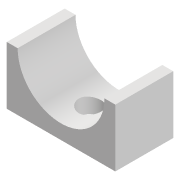
# Autodesk Inventor part: Tube_adaptor_2
Saved by Autodesk Inventor 2022 (Build 260153000, 153)
## iProperties
Created: 2022-06-09
Part Number: Tube_adaptor_2
Material: Generic
Document SubType Name: Modeling
Designer: dell
Density: 1 g/cm^3
Appearance: Default
Author: dell
Autodesk Inventor part; units mm, degrees
ref_plane "YZ Plane" through (0, 0, 0) normal (1, 0, 0) x (0, 1, 0)
ref_plane "XZ Plane" through (0, 0, 0) normal (0, 1, 0) x (-1, 0, 0)
ref_plane "XY Plane" through (0, 0, 0) normal (0, 0, 1) x (1, 0, 0)
sketch "Sketch1" plane through (0, 0, 0) normal (0, 0, 1) x (1, 0, 0)
  circle A0 centre (0, 0) radius 6
  line L0 (-7.5, 0) -> (7.5, 0)
  line L1 (7.5, 0) -> (7.5, -8)
  line L2 (7.5, -8) -> (-7.5, -8)
  line L3 (-7.5, -8) -> (-7.5, 0)
  point P0 (6, 0)
  point P1 (-6, 0)
  point P2 (6, 0)
  point P3 (-6, 0)
  dimension "d0" = 12
  dimension "d1" = 2
  dimension "d2" = 7.5
  dimension "d3" = 7.5
  constraints: 8 end point, 2 parallel, 1 centre point, 1 coincident, 1 horizontal, 1 midpoint, 1 perpendicular
  measures "d0" diameter of A0
  measures "d1" distance edge to line of A0 L2
  measures "d2" distance from line of point (0, 0) L1
  measures "d3" distance from line of point (0, 0) L3
extrude "Extrusion1" add sketch "Sketch1" along normal blind 8 contours L0 L1 L2 L3 A0
sketch "Sketch2" plane through (-7.5, -8, 0) normal (0, -1, 0) x (1, 0, 0)
  line L0 (0, 0) -> (15, 0) projected
  line L1 (15, 0) -> (15, 8) projected
  line L2 (0, 8) -> (15, 8) projected
  line L3 (0, 0) -> (0, 8) projected
  line L4 (0, 8) -> (15, 8) construction
  line L5 (15, 0) -> (0, 8) construction
  line L6 (0, 0) -> (15, 0) construction
  line L7 (15, 8) -> (0, 0) construction
  circle A0 centre (7.5, 4) radius 1.55
  point P0 (7.5, 0)
  dimension "d6" = 3.1
  constraints: 4 end point, 1 centre point, 1 midpoint
  measures "d6" diameter of A0
extrude "Extrusion2" cut sketch "Sketch2" along normal mid plane 6 contours A0
body "Solid1"
